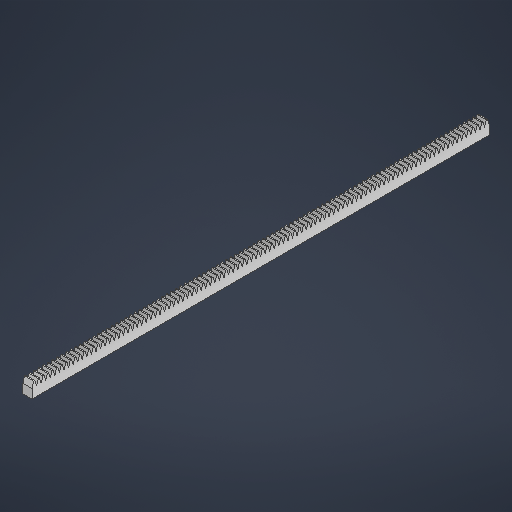
# Autodesk Inventor part: Rack
Saved by Autodesk Inventor 2026.1 (Build 301233020, 233B)
## iProperties
Created: 2026-03-11
Part Number: Rack
Material: Generic
Document SubType Name: Modeling
Designer: elaij
Density: 1 g/cm^3
Appearance: Default
Author: elaij
Autodesk Inventor part; units mm, degrees
ref_plane "YZ Plane" through (0, 0, 0) normal (1, 0, 0) x (0, 1, 0)
ref_plane "XZ Plane" through (0, 0, 0) normal (0, 1, 0) x (-1, 0, 0)
ref_plane "XY Plane" through (0, 0, 0) normal (0, 0, 1) x (1, 0, 0)
sketch "Sketch1" plane through (0, 0, 0) normal (1, 0, 0) x (0, 1, 0)
  line L0 (0, 0) -> (10, 0)
  line L1 (10, 0) -> (10, 500)
  line L2 (10, 500) -> (0, 500)
  line L3 (0, 500) -> (0, 0)
  line L4 (10, 0) -> (18, 2.5)
  line L5 (18, 2.5) -> (10, 2.5)
  line L6 (10, 5) -> (18, 2.5)
  line L7 (18, 0) -> (18, 2.5)
  line L8 (10, 5) -> (18, 7.5)
  line L9 (10, 10) -> (18, 7.5)
  line L10 (10, 10) -> (18, 12.5)
  line L11 (10, 15) -> (18, 12.5)
  line L12 (10, 15) -> (18, 17.5)
  line L13 (10, 20) -> (18, 17.5)
  line L14 (10, 20) -> (18, 22.5)
  line L15 (10, 25) -> (18, 22.5)
  line L16 (10, 25) -> (18, 27.5)
  line L17 (10, 30) -> (18, 27.5)
  line L18 (10, 30) -> (18, 32.5)
  line L19 (10, 35) -> (18, 32.5)
  line L20 (10, 35) -> (18, 37.5)
  line L21 (10, 40) -> (18, 37.5)
  line L22 (10, 40) -> (18, 42.5)
  line L23 (10, 45) -> (18, 42.5)
  line L24 (10, 45) -> (18, 47.5)
  line L25 (10, 50) -> (18, 47.5)
  line L26 (10, 50) -> (18, 52.5)
  line L27 (10, 55) -> (18, 52.5)
  line L28 (10, 55) -> (18, 57.5)
  line L29 (10, 60) -> (18, 57.5)
  line L30 (10, 60) -> (18, 62.5)
  line L31 (10, 65) -> (18, 62.5)
  line L32 (10, 65) -> (18, 67.5)
  line L33 (10, 70) -> (18, 67.5)
  line L34 (10, 70) -> (18, 72.5)
  line L35 (10, 75) -> (18, 72.5)
  line L36 (10, 75) -> (18, 77.5)
  line L37 (10, 80) -> (18, 77.5)
  line L38 (10, 80) -> (18, 82.5)
  line L39 (10, 85) -> (18, 82.5)
  line L40 (10, 85) -> (18, 87.5)
  line L41 (10, 90) -> (18, 87.5)
  line L42 (10, 90) -> (18, 92.5)
  line L43 (10, 95) -> (18, 92.5)
  line L44 (10, 95) -> (18, 97.5)
  line L45 (10, 100) -> (18, 97.5)
  line L46 (10, 100) -> (18, 102.5)
  line L47 (10, 105) -> (18, 102.5)
  line L48 (10, 105) -> (18, 107.5)
  line L49 (10, 110) -> (18, 107.5)
  line L50 (10, 110) -> (18, 112.5)
  line L51 (10, 115) -> (18, 112.5)
  line L52 (10, 115) -> (18, 117.5)
  line L53 (10, 120) -> (18, 117.5)
  line L54 (10, 120) -> (18, 122.5)
  line L55 (10, 125) -> (18, 122.5)
  line L56 (10, 125) -> (18, 127.5)
  line L57 (10, 130) -> (18, 127.5)
  line L58 (10, 130) -> (18, 132.5)
  line L59 (10, 135) -> (18, 132.5)
  line L60 (10, 135) -> (18, 137.5)
  line L61 (10, 140) -> (18, 137.5)
  line L62 (10, 140) -> (18, 142.5)
  line L63 (10, 145) -> (18, 142.5)
  line L64 (10, 145) -> (18, 147.5)
  line L65 (10, 150) -> (18, 147.5)
  line L66 (10, 150) -> (18, 152.5)
  line L67 (10, 155) -> (18, 152.5)
  line L68 (10, 155) -> (18, 157.5)
  line L69 (10, 160) -> (18, 157.5)
  line L70 (10, 160) -> (18, 162.5)
  line L71 (10, 165) -> (18, 162.5)
  line L72 (10, 165) -> (18, 167.5)
  line L73 (10, 170) -> (18, 167.5)
  line L74 (10, 170) -> (18, 172.5)
  line L75 (10, 175) -> (18, 172.5)
  line L76 (10, 175) -> (18, 177.5)
  line L77 (10, 180) -> (18, 177.5)
  line L78 (10, 180) -> (18, 182.5)
  line L79 (10, 185) -> (18, 182.5)
  line L80 (10, 185) -> (18, 187.5)
  line L81 (10, 190) -> (18, 187.5)
  line L82 (10, 190) -> (18, 192.5)
  line L83 (10, 195) -> (18, 192.5)
  line L84 (10, 195) -> (18, 197.5)
  line L85 (10, 200) -> (18, 197.5)
  line L86 (10, 200) -> (18, 202.5)
  line L87 (10, 205) -> (18, 202.5)
  line L88 (10, 205) -> (18, 207.5)
  line L89 (10, 210) -> (18, 207.5)
  line L90 (10, 210) -> (18, 212.5)
  line L91 (10, 215) -> (18, 212.5)
  line L92 (10, 215) -> (18, 217.5)
  line L93 (10, 220) -> (18, 217.5)
  line L94 (10, 220) -> (18, 222.5)
  line L95 (10, 225) -> (18, 222.5)
  line L96 (10, 225) -> (18, 227.5)
  line L97 (10, 230) -> (18, 227.5)
  line L98 (10, 230) -> (18, 232.5)
  line L99 (10, 235) -> (18, 232.5)
  line L100 (10, 235) -> (18, 237.5)
  line L101 (10, 240) -> (18, 237.5)
  line L102 (10, 240) -> (18, 242.5)
  line L103 (10, 245) -> (18, 242.5)
  line L104 (10, 245) -> (18, 247.5)
  line L105 (10, 250) -> (18, 247.5)
  line L106 (10, 250) -> (18, 252.5)
  line L107 (10, 255) -> (18, 252.5)
  line L108 (10, 255) -> (18, 257.5)
  line L109 (10, 260) -> (18, 257.5)
  line L110 (10, 260) -> (18, 262.5)
  line L111 (10, 265) -> (18, 262.5)
  line L112 (10, 265) -> (18, 267.5)
  line L113 (10, 270) -> (18, 267.5)
  line L114 (10, 270) -> (18, 272.5)
  line L115 (10, 275) -> (18, 272.5)
  line L116 (10, 275) -> (18, 277.5)
  line L117 (10, 280) -> (18, 277.5)
  line L118 (10, 280) -> (18, 282.5)
  line L119 (10, 285) -> (18, 282.5)
  line L120 (10, 285) -> (18, 287.5)
  line L121 (10, 290) -> (18, 287.5)
  line L122 (10, 290) -> (18, 292.5)
  line L123 (10, 295) -> (18, 292.5)
  line L124 (10, 295) -> (18, 297.5)
  line L125 (10, 300) -> (18, 297.5)
  line L126 (10, 300) -> (18, 302.5)
  line L127 (10, 305) -> (18, 302.5)
  line L128 (10, 305) -> (18, 307.5)
  line L129 (10, 310) -> (18, 307.5)
  line L130 (10, 310) -> (18, 312.5)
  line L131 (10, 315) -> (18, 312.5)
  line L132 (10, 315) -> (18, 317.5)
  line L133 (10, 320) -> (18, 317.5)
  line L134 (10, 320) -> (18, 322.5)
  line L135 (10, 325) -> (18, 322.5)
  line L136 (10, 325) -> (18, 327.5)
  line L137 (10, 330) -> (18, 327.5)
  line L138 (10, 330) -> (18, 332.5)
  line L139 (10, 335) -> (18, 332.5)
  line L140 (10, 335) -> (18, 337.5)
  line L141 (10, 340) -> (18, 337.5)
  line L142 (10, 340) -> (18, 342.5)
  line L143 (10, 345) -> (18, 342.5)
  line L144 (10, 345) -> (18, 347.5)
  line L145 (10, 350) -> (18, 347.5)
  line L146 (10, 350) -> (18, 352.5)
  line L147 (10, 355) -> (18, 352.5)
  line L148 (10, 355) -> (18, 357.5)
  line L149 (10, 360) -> (18, 357.5)
  line L150 (10, 360) -> (18, 362.5)
  line L151 (10, 365) -> (18, 362.5)
  line L152 (10, 365) -> (18, 367.5)
  line L153 (10, 370) -> (18, 367.5)
  line L154 (10, 370) -> (18, 372.5)
  line L155 (10, 375) -> (18, 372.5)
  line L156 (10, 375) -> (18, 377.5)
  line L157 (10, 380) -> (18, 377.5)
  line L158 (10, 380) -> (18, 382.5)
  line L159 (10, 385) -> (18, 382.5)
  line L160 (10, 385) -> (18, 387.5)
  line L161 (10, 390) -> (18, 387.5)
  line L162 (10, 390) -> (18, 392.5)
  line L163 (10, 395) -> (18, 392.5)
  line L164 (10, 395) -> (18, 397.5)
  line L165 (10, 400) -> (18, 397.5)
  line L166 (10, 400) -> (18, 402.5)
  line L167 (10, 405) -> (18, 402.5)
  line L168 (10, 405) -> (18, 407.5)
  line L169 (10, 410) -> (18, 407.5)
  line L170 (10, 410) -> (18, 412.5)
  line L171 (10, 415) -> (18, 412.5)
  line L172 (10, 415) -> (18, 417.5)
  line L173 (10, 420) -> (18, 417.5)
  line L174 (10, 420) -> (18, 422.5)
  line L175 (10, 425) -> (18, 422.5)
  line L176 (10, 425) -> (18, 427.5)
  line L177 (10, 430) -> (18, 427.5)
  line L178 (10, 430) -> (18, 432.5)
  line L179 (10, 435) -> (18, 432.5)
  line L180 (10, 435) -> (18, 437.5)
  line L181 (10, 440) -> (18, 437.5)
  line L182 (10, 440) -> (18, 442.5)
  line L183 (10, 445) -> (18, 442.5)
  line L184 (10, 445) -> (18, 447.5)
  line L185 (10, 450) -> (18, 447.5)
  line L186 (10, 450) -> (18, 452.5)
  line L187 (10, 455) -> (18, 452.5)
  line L188 (10, 455) -> (18, 457.5)
  line L189 (10, 460) -> (18, 457.5)
  line L190 (10, 460) -> (18, 462.5)
  line L191 (10, 465) -> (18, 462.5)
  line L192 (10, 465) -> (18, 467.5)
  line L193 (10, 470) -> (18, 467.5)
  line L194 (10, 470) -> (18, 472.5)
  line L195 (10, 475) -> (18, 472.5)
  line L196 (10, 475) -> (18, 477.5)
  line L197 (10, 480) -> (18, 477.5)
  line L198 (10, 480) -> (18, 482.5)
  line L199 (10, 485) -> (18, 482.5)
  line L200 (10, 485) -> (18, 487.5)
  line L201 (10, 490) -> (18, 487.5)
  line L202 (10, 490) -> (18, 492.5)
  line L203 (10, 495) -> (18, 492.5)
  line L204 (10, 495) -> (18, 497.5)
  line L205 (10, 500) -> (18, 497.5)
  dimension "d1" = 10
  dimension "d2" = 5
  dimension "d3" = 500
  dimension "d5" = 8
  dimension "d18" = 5
  constraints: 410 end point, 297 vertical alignment, 199 parallel, 3 horizontal, 1 perpendicular, 1 symmetric about line, 1 vertical, 3 other
  measures "d2" distance of L6.start L0.end
  measures "d3" distance between parallel lines of L2 L0
  measures "d18" distance of L0.end L8.start
extrude "Extrusion1" add sketch "Sketch1" along normal blind 10
sketch "Sketch2" plane through (10, 0, 0) normal (1, 0, 0) x (0, 0, -1)
  line L0 (-2.5, 18) -> (-5, 10) projected
  line L1 (0, 18) -> (-500, 18)
  line L2 (-500, 18) -> (-500, 16)
  line L3 (-500, 16) -> (0, 16)
  line L4 (0, 16) -> (0, 18)
  point P0 (0, 0)
  point P1 (0, 17)
  point P2 (0, 10)
  dimension "d25" = 500
  dimension "d26" = 8
  dimension "d27" = 2
  constraints: 8 end point, 2 parallel, 1 horizontal, 1 midpoint, 1 perpendicular, 1 vertical alignment
  measures "d25" distance of L1.start L1.end
  measures "d26" distance from line of L0.end L1
  measures "d27" distance between parallel lines of L1 L3
extrude "Extrusion2" cut sketch "Sketch2" against normal blind 10
equation "\"d2\" = Pitch"
equation "\"d3\" = Length"
equation "\"d5\" = ToothHeight"
equation "\"d18\" = Pitch"
equation "\"d23\" = Width"
equation "\"d25\" = Length"
equation "\"d26\" = ToothHeight"
equation "\"d27\" = ToothCut"
equation "\"d28\" = Width"
equation "\"Length\" = 500"
equation "\"Pitch\" = 5"
equation "\"ToothHeight\" = 8"
equation "\"ToothCut\" = 2"
equation "\"Width\" = 10"
body "Solid1"
